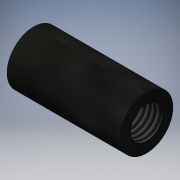
# Autodesk Inventor part: dc cover
Saved by Autodesk Inventor 2019 (Build 230136000, 136)
## iProperties
Created: 2020-03-05
Part Number: dc cover
Material: Generic
Document SubType Name: Modeling
Designer: ntb11189
Density: 1 g/cm^3
Appearance: Smooth - Black
Author: ntb11189
Autodesk Inventor part; units mm, degrees
ref_plane "YZ Plane" through (0, 0, 0) normal (1, 0, 0) x (0, 1, 0)
ref_plane "XZ Plane" through (0, 0, 0) normal (0, 1, 0) x (-1, 0, 0)
ref_plane "XY Plane" through (0, 0, 0) normal (0, 0, 1) x (1, 0, 0)
sketch "Sketch1" plane through (0, 0, 0) normal (1, 0, 0) x (0, 1, 0)
  circle A0 centre (0, 0) radius 4.25
  circle A1 centre (0, 0) radius 2.5
  dimension "d0" = 4.25
  dimension "d3" = 2.5
  constraints: 2 centre point, 2 coincident
  measures "d0" radius of A0
  measures "d3" radius of A1
extrude "Extrusion2" add sketch "Sketch1" along normal blind 18
thread "Thread1" size "M5x0.8" class "6H" standard "ANSI Metric M Profile" length 5
body "Solid2"
